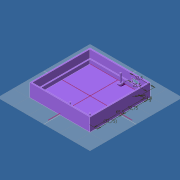
# Autodesk Inventor part: Sensorlamp_Base_new
Saved by Autodesk Inventor 2016 SP2 (Build 200236200, 236)
## iProperties
Created: 2017-11-09
Part Number: Sensorlamp_Base_new
Material: Generisch
Document SubType Name: Modeling
Designer: User
Density: 1 g/cm^3
Appearance: Violett
Author: User
Autodesk Inventor part; units mm, degrees
ref_plane "YZ Plane" through (0, 0, 0) normal (1, 0, 0) x (0, 1, 0)
ref_plane "XZ Plane" through (0, 0, 0) normal (0, 1, 0) x (-1, 0, 0)
ref_plane "XY Plane" through (0, 0, 0) normal (0, 0, 1) x (1, 0, 0)
sketch "USB_Micro" plane through (0, 0, 0) normal (0, 0, 1) x (1, 0, 0)
  line L0 (-6.7, 3.4) -> (-6.7, 2.0438)
  line L1 (-7.2, 1.6938) -> (-6.7, 2.0438)
  line L2 (-7.2, 1.6938) -> (-7.2, 0.3)
  line L3 (-7.2, 0.3) -> (-0.3, 0.3)
  line L4 (-0.3, 0.3) -> (-0.3, 1.6938)
  line L5 (-0.8, 2.0438) -> (-0.3, 1.6938)
  line L6 (-6.7, 3.4) -> (-0.8, 3.4)
  line L7 (-0.8, 3.4) -> (-0.8, 2.0438)
  line L8 (-0.8, 0.8) -> (-6.7, 0.8)
  line L9 (-6.7, 0.8) -> (-6.7, 1.4335)
  line L10 (-6.7, 1.4335) -> (-6.2, 1.7835)
  line L11 (-6.2, 1.7835) -> (-6.2, 2.9)
  line L12 (-6.2, 2.9) -> (-1.3, 2.9)
  line L13 (-1.3, 2.9) -> (-1.3, 1.7835)
  line L14 (-1.3, 1.7835) -> (-0.8, 1.4335)
  line L15 (-0.8, 1.4335) -> (-0.8, 0.8)
  point P0 (-3.75, 0.3)
  dimension "d42" = 0.5
  measures "d42" distance between parallel lines of L3 L8
sketch "Skizze1" plane through (0, 0, 0) normal (0, 0, 1) x (1, 0, 0)
  line L0 (-39, -39) -> (39, -39)
  line L1 (39, -39) -> (39, 39)
  line L2 (39, 39) -> (-39, 39)
  line L3 (-39, 39) -> (-39, -39)
  line L4 (-39, -39) -> (39, 39) construction
  line L5 (39, -39) -> (-39, 39) construction
  line L6 (-37.5, -37.5) -> (37.5, -37.5)
  line L7 (37.5, -37.5) -> (37.5, 37.5)
  line L8 (37.5, 37.5) -> (-37.5, 37.5)
  line L9 (-37.5, 37.5) -> (-37.5, -37.5)
  line L10 (-37.5, -37.5) -> (37.5, 37.5) construction
  line L11 (37.5, -37.5) -> (-37.5, 37.5) construction
  line L12 (-37.5, 37.5) -> (-36, 37.5)
  line L13 (-36, 37.5) -> (-36, -37.5)
  line L14 (-36, -37.5) -> (-37.5, -37.5)
  line L15 (-37.5, -37.5) -> (-37.5, 37.5)
  line L16 (36, 37.5) -> (37.5, 37.5)
  line L17 (37.5, 37.5) -> (37.5, -37.5)
  line L18 (37.5, -37.5) -> (36, -37.5)
  line L19 (36, -37.5) -> (36, 37.5)
  line L20 (-36, -36) -> (36, -36)
  line L21 (36, -36) -> (36, -37.5)
  line L22 (36, -37.5) -> (-36, -37.5)
  line L23 (-36, -37.5) -> (-36, -36)
  line L24 (36, 37.5) -> (-36, 37.5)
  line L25 (-36, 37.5) -> (-36, 36)
  line L26 (-36, 36) -> (36, 36)
  line L27 (36, 36) -> (36, 37.5)
  point P0 (0, 0)
  dimension "d0" = 78
  dimension "d1" = 78
  dimension "d2" = 75
  dimension "d3" = 75
  dimension "d46" = 1.5
  dimension "d47" = 1.5
  dimension "d48" = 1.5
  dimension "d52" = 1.5
  constraints: 56 end point, 12 parallel, 6 horizontal, 6 perpendicular, 4 midpoint, 4 point on line
  measures "d0" distance of L1.end L2.end
  measures "d1" distance of L2.end L0.start
  measures "d2" distance of L8.end L7.end
  measures "d3" distance of L7.end L6.end
  measures "d46" distance between parallel lines of L15 L13
  measures "d47" distance between parallel lines of L17 L19
  measures "d48" distance between parallel lines of L22 L20
  measures "d52" distance between parallel lines of L26 L24
extrude "Extrusion1" add sketch "Skizze1" along normal blind 15
extrude "Extrusion9" add sketch "Skizze1" along normal blind 5 contours L9 L8 L13 L6 | L13 L20 L19 L6 | L19 L8 L7 L6 | L8 L19 L26 L13
extrude "Extrusion6" add sketch "Skizze1" against normal blind 2 contours L3 L2 L1 L0 | L9 L8 L13 L6 | L13 L20 L19 L6 | L19 L8 L7 L6 | L13 L26 L19 L20 | L8 L19 L26 L13
sketch "Skizze5" plane through (0, 0, 0) normal (0, 0, 1) x (1, 0, 0)
  circle A0 centre (32.5, -32.75) radius 0.9
  circle A1 centre (32.5, 32.75) radius 0.9
  circle A2 centre (7, -32.75) radius 0.9
  circle A3 centre (7, 32.75) radius 0.9
  circle A4 centre (32.5, 32.75) radius 2.5
  circle A5 centre (7, 32.75) radius 2.5
  circle A6 centre (32.5, -32.75) radius 2.5
  circle A7 centre (7, -32.75) radius 2.5
  line L0 (-54.6, 0) -> (54.6, 0) projected
  line L1 (0, -54.6) -> (0, 54.6) projected
  line L2 (36, 36) -> (36, -36) projected
  line L3 (-36, 36) -> (36, 36) projected
  line L4 (36, -36) -> (-36, -36) projected
  line L5 (9.5, 32.75) -> (9.5, 36)
  line L6 (4.5, 32.75) -> (4.5, 36)
  line L7 (4.5, 36) -> (9.5, 36)
  line L8 (30, 32.75) -> (30, 36)
  line L9 (30, 36) -> (36, 36)
  line L10 (32.5, 30.25) -> (36, 30.25)
  line L11 (36, 30.25) -> (36, 36)
  line L12 (32.5, -30.25) -> (36, -30.25)
  line L13 (36, -30.25) -> (36, -36)
  line L14 (30, -32.75) -> (30, -36)
  line L15 (30, -36) -> (36, -36)
  line L16 (9.5, -32.75) -> (9.5, -36)
  line L17 (4.5, -32.75) -> (4.5, -36)
  line L18 (4.5, -36) -> (9.5, -36)
  point P0 (0, 0)
  dimension "d28" = 1.8
  dimension "d33" = 5
  dimension "d34" = 65.5
  dimension "d35" = 25.5
  dimension "d36" = 32.5
  dimension "d37" = 32.75
  dimension "d51" = 32.75
  constraints: 28 end point, 9 perpendicular, 8 centre point, 8 point on circle, 8 point on line, 8 tangent, 6 equal radius, 4 coincident, 4 collinear, 2 horizontal alignment, 2 vertical alignment, 1 horizontal
  measures "d28" diameter of A1
  measures "d33" diameter of A4
  measures "d34" distance of A0.centre A1.centre
  measures "d35" distance of A3.centre A1.centre
  measures "d36" distance from line of L1 A1.centre
  measures "d37" distance from line of L0 A1.centre
  measures "d51" distance from line of L0 A0.centre
extrude "Extrusion7" add sketch "Skizze5" along normal blind 2 contours A4 | A5 | A6 | A7
sketch "Skizze6" plane through (-39, 39, 15) normal (0, 1, 0) x (1, 0, 0)
  line L0 (63.71, 5.7) -> (56.21, 5.7) projected
  line L1 (63.71, 7.55) -> (63.71, 5.7) projected
  line L2 (63.71, 7.55) -> (63.21, 7.9) projected
  line L3 (63.21, 7.9) -> (63.21, 9.4) projected
  line L4 (56.71, 9.4) -> (63.21, 9.4) projected
  line L5 (56.71, 7.9) -> (56.71, 9.4) projected
  line L6 (56.21, 7.55) -> (56.71, 7.9) projected
  line L7 (56.21, 7.55) -> (56.21, 5.7) projected
  line L8 (56.51, 6) -> (63.41, 6) projected
  line L9 (56.51, 7.3938) -> (56.51, 6) projected
  line L10 (57.01, 7.7438) -> (56.51, 7.3938) projected
  line L11 (57.01, 9.1) -> (57.01, 7.7438) projected
  line L12 (62.91, 9.1) -> (57.01, 9.1) projected
  line L13 (62.91, 9.1) -> (62.91, 7.7438) projected
  line L14 (62.91, 7.7438) -> (63.41, 7.3938) projected
  line L15 (63.41, 7.3938) -> (63.41, 6) projected
  line L16 (64.46, 4.95) -> (55.46, 4.95)
  line L17 (55.46, 4.95) -> (55.46, 7.9405)
  line L18 (55.46, 7.9405) -> (55.96, 8.2905)
  line L19 (55.96, 8.2905) -> (55.96, 10.15)
  line L20 (55.96, 10.15) -> (63.96, 10.15)
  line L21 (63.96, 10.15) -> (63.96, 8.2905)
  line L22 (63.96, 8.2905) -> (64.46, 7.9405)
  line L23 (64.46, 7.9405) -> (64.46, 4.95)
  point P0 (39, 15)
  dimension "d45" = 0.75
  constraints: 16 end point, 7 other
  measures "d45" distance between parallel lines of L1 L23
extrude "Extrusion8" cut sketch "Skizze6" against normal up to surface (3 mm away) contours L0 L7 L6 L5 L4 L3 L2 L1 | L9 L10 L11 L12 L13 L14 L15 L8 | L16 L17 L18 L19 L20 L21 L22 L23
extrude "Extrusion10" add sketch "Skizze5" along normal blind 13 contours A0 | A1 | A2 | A3
equation "\"d0\" = d1"
equation "\"d2\" = d3"
equation "\"d47\" = d46"
equation "\"d48\" = d46"
equation "\"d52\" = d46"
